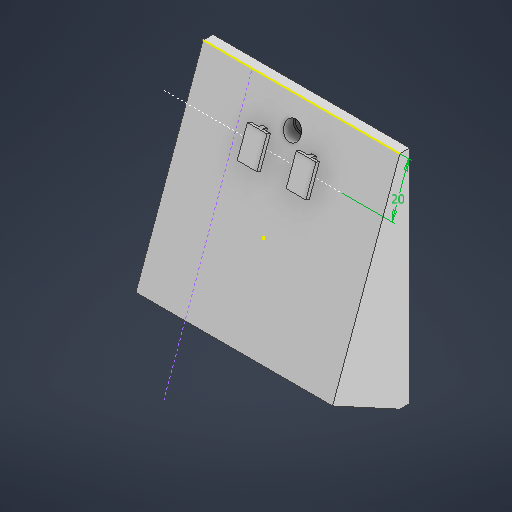
# Autodesk Inventor part: LCD_Mount_20degrees
Saved by Autodesk Inventor 2026.2 (Build 302298010, 298A)
## iProperties
Created: 2026-08-14
Part Number: LCD_Mount_20degrees
Material: 일반
Document SubType Name: Modeling
Designer: User
Density: 1 g/cm^3
Appearance: 기본값
Author: User
Autodesk Inventor part; units mm, degrees
ref_plane "YZ Plane" through (0, 0, 0) normal (1, 0, 0) x (0, 1, 0)
sketch "스케치2" plane through (0, 0, 0) normal (1, 0, 0) x (0, 1, 0)
  line L0 (-42.3529, 0) -> (47.6471, 0) construction
  line L1 (47.6471, 0) -> (-27.5284, 27.3616)
  line L2 (-27.5284, 27.3616) -> (-42.3529, 0)
  line L3 (47.6471, 0) -> (-42.3529, 0) construction
  line L4 (-42.3529, 0) -> (-42.3529, -4)
  line L5 (-42.3529, -4) -> (47.6471, -4)
  line L6 (47.6471, -4) -> (47.6471, 0)
  point P0 (0, 0)
  dimension "d2" = 90
  dimension "d3" = 80
  dimension "d4" = 20
  dimension "d7" = 4
  constraints: 14 end point, 2 horizontal, 2 parallel, 1 perpendicular
  measures "d2" distance of L0.start L0.end
  measures "d3" distance of L0.end L1.end
  measures "d4" angle of L0 L1
  measures "d7" distance of L3.end L4.end
extrude "돌출2" add sketch "스케치2" along normal mid plane 80
sketch "스케치3" plane through (40, 47.6471, -4) normal (0, 0, -1) x (-1, 0, 0)
  line L0 (80, 0) -> (0, 0) projected
  line L1 (0, -10) -> (40, -10)
  line L2 (80, -90) -> (0, -90) projected
  line L3 (0, -75.1754) -> (0, -90) projected
  line L4 (0, -80) -> (80, -80)
  line L5 (80, 0) -> (80, -90) projected
  line L6 (40, -93) -> (40, 7) construction
  circle A0 centre (40, -80) radius 2.5
  circle A1 centre (40, -10) radius 2.5
  line L7 (0, 0) -> (0, -75.1754) projected
  point P0 (40, -47.6471)
  dimension "d10" = 10
  dimension "d12" = 10
  dimension "d13" = 5
  dimension "d14" = 5
  dimension "d44" = 40
  constraints: 6 end point, 4 point on line, 2 centre point, 2 horizontal, 1 midpoint, 1 vertical, 2 other
  measures "d10" distance between parallel lines of L1 L0
  measures "d12" distance between parallel lines of L2 L4
  measures "d13" diameter of A0
  measures "d14" diameter of A1
  measures "d44" distance between parallel lines of L7 L6
extrude "돌출3" cut sketch "스케치3" against normal blind 40 contours A1 | A0 L4 | L4 A0
ref_plane "작업 평면3" through (0, 0, 27) normal (0, 0, 1) x (1, 0, 0)
sketch "스케치4" plane through (0, 0, 27) normal (0, 0, 1) x (1, 0, 0)
  circle A0 centre (0, 37.6471) radius 2.5 projected
  circle A1 centre (0, -32.3529) radius 2.5 projected
  circle A2 centre (0, 37.6471) radius 3.5
  circle A3 centre (0, -32.3529) radius 3.5
  point P0 (0, 0)
  dimension "d18" = 7
  dimension "d19" = 7
  constraints: 2 centre point, 2 coincident
  measures "d18" diameter of A2
  measures "d19" diameter of A3
extrude "돌출4" cut sketch "스케치4" against normal blind 27 contours A0 | A1 | A2 | A3
sketch "스케치5" plane through (-40, -27.5284, 27.3616) normal (0, 0.342, 0.9397) x (1, 0, 0)
  line L0 (20, 80) -> (20, -25) construction
  line L1 (-10, 60) -> (63, 60) construction
  line L2 (0, 80) -> (80, 80) projected
  point P0 (40, 35.2264)
  dimension "d22" = 20
  constraints: 4 end point, 1 horizontal, 1 vertical
  measures "d22" distance between parallel lines of L1 L2
ref_plane "작업 평면4" through (-50, 28.8532, 6.8404) normal (0, -0.9397, 0.342) x (1, 0, 0)
sketch "스케치6" plane through (-50, 28.8532, 6.8404) normal (0, -0.9397, 0.342) x (1, 0, 0)
  line L0 (50, 15) -> (50, -51) construction
  line L1 (46.5, 0) -> (53.5, 0) projected
  line L2 (10, 0) -> (90, 0) projected
  line L3 (21, 0) -> (21, 0)
  line L4 (90, 0) -> (90, -30.7818) projected
  line L5 (39.1, 0) -> (41, 0)
  line L6 (41, 0) -> (41, 2)
  line L7 (39.1, 2) -> (39.1, 0)
  line L8 (36.05, 3.5) -> (44.05, 3.5)
  line L9 (44.05, 3.5) -> (44.05, 2)
  line L10 (36.05, 2) -> (36.05, 3.5)
  line L11 (44.05, 2) -> (41, 2)
  line L12 (39.1, 2) -> (36.05, 2)
  line L13 (59, 0) -> (59, 2)
  line L14 (60.9, 2) -> (60.9, 0)
  line L15 (63.95, 3.5) -> (55.95, 3.5)
  line L16 (55.95, 3.5) -> (55.95, 2)
  line L17 (63.95, 2) -> (63.95, 3.5)
  line L18 (55.95, 2) -> (59, 2)
  line L19 (60.9, 2) -> (63.95, 2)
  line L20 (10, -30.7818) -> (10, 0) projected
  point P0 (50, -16.2963)
  point P1 (41, 1)
  point P2 (59, 1)
  point P3 (59, 0)
  point P4 (60.9, 0)
  dimension "d30" = 9
  dimension "d35" = 8
  dimension "d36" = 1.5
  dimension "d37" = 2
  dimension "d38" = 3.05
  dimension "d41" = 1.5
  dimension "d42" = 3.05
  dimension "d43" = 40
  constraints: 34 end point, 9 symmetric about line, 4 parallel, 3 horizontal, 2 perpendicular, 2 point on line, 1 midpoint, 1 vertical
  measures "d30" distance from line of L0 point (41, 1)
  measures "d35" distance of L8.start L8.end
  measures "d36" distance of L10.start L8.start
  measures "d37" distance of L7.start L5.start
  measures "d38" distance of L7.start L10.start
  measures "d41" distance of L8.end L9.end
  measures "d42" distance between parallel lines of L6 L9
  measures "d43" distance between parallel lines of L20 L0
extrude "돌출5" add sketch "스케치6" along normal mid plane 12
